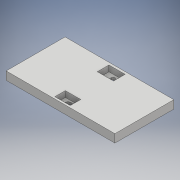
# Autodesk Inventor part: Parte7
Saved by Autodesk Inventor 2017 (Build 210142000, 142)
## iProperties
Part Number: Parte7
Material: Generico
Document SubType Name: Modeling
Designer: Federico
Density: 1 g/cm^3
Appearance: Default
Author: Federico
Autodesk Inventor part; units mm, degrees
ref_plane "YZ Plane" through (0, 0, 0) normal (1, 0, 0) x (0, 1, 0)
ref_plane "XZ Plane" through (0, 0, 0) normal (0, 1, 0) x (-1, 0, 0)
ref_plane "XY Plane" through (0, 0, 0) normal (0, 0, 1) x (1, 0, 0)
sketch "Schizzo1" plane through (0, 0, 0) normal (0, 0, 1) x (1, 0, 0)
  line L0 (-60, 32.5) -> (60, 32.5)
  line L1 (60, 32.5) -> (60, -32.5)
  line L2 (60, -32.5) -> (-60, -32.5)
  line L3 (-60, -32.5) -> (-60, 32.5)
  line L4 (-60, 32.5) -> (60, -32.5) construction
  line L5 (60, 32.5) -> (-60, -32.5) construction
  line L6 (-8.5, -18.7) -> (8.5, -18.7)
  line L7 (8.5, -18.7) -> (8.5, -30.3)
  line L8 (8.5, -30.3) -> (-8.5, -30.3)
  line L9 (-8.5, -30.3) -> (-8.5, -18.7)
  line L10 (-8.5, -18.7) -> (8.5, -30.3) construction
  line L11 (8.5, -18.7) -> (-8.5, -30.3) construction
  line L12 (-12, 12) -> (12, -12) construction
  line L13 (12, 12) -> (-12, -12) construction
  line L14 (-8.95, 29.85) -> (8.95, 29.85)
  line L15 (8.95, 29.85) -> (8.95, 17)
  line L16 (8.95, 17) -> (-8.95, 17)
  line L17 (-8.95, 17) -> (-8.95, 29.85)
  line L18 (-8.95, 29.85) -> (8.95, 17) construction
  line L19 (8.95, 29.85) -> (-8.95, 17) construction
  circle A0 centre (0, -24.5) radius 4.1
  line L20 (0, 25.425) -> (0, 21.425) construction
  line L21 (-2, 25.425) -> (-2, 21.425)
  line L22 (2, 21.425) -> (2, 25.425)
  arc A1 (2, 25.425) -> (-2, 25.425) centre (0, 25.425) ccw
  arc A2 (-2, 21.425) -> (2, 21.425) centre (0, 21.425) ccw
  point P0 (0, 0)
  point P1 (0, 0)
  point P2 (0, 23.425)
  dimension "d0" = 120
  dimension "d1" = 65
  dimension "d2" = 17
  dimension "d3" = 11.6
  dimension "d4" = 24
  dimension "d5" = 24
  dimension "d6" = 17.9
  dimension "d7" = 12.85
  dimension "d8" = 8.2
  dimension "d9" = 2
  dimension "d10" = 4
  constraints: 48 end point, 7 midpoint, 7 parallel, 4 perpendicular, 4 point on circle, 4 tangent, 3 centre point, 3 horizontal
  measures "d0" distance of L1.end L2.end
  measures "d1" distance of L0.end L1.end
  measures "d2" distance of L7.end L8.end
  measures "d3" distance of L6.end L7.end
  measures "d4" distance of L12.end L13.end
  measures "d5" distance of L13.start L12.end
  measures "d6" distance of L16.start L17.start
  measures "d7" distance of L14.end L16.start
  measures "d8" diameter of A0
  measures "d9" distance of point (0, 23.425) L20.end
  measures "d10" diameter of A2
extrude "Estrusione1" add sketch "Schizzo1" along normal blind 9 contours L0 L1 L2 L3
sketch "Schizzo2" plane through (0, 0, 0) normal (0, 0, -1) x (-1, 0, 0)
  line L0 (-60, 32.5) -> (60, 32.5)
  line L1 (60, 32.5) -> (60, -32.5)
  line L2 (60, -32.5) -> (-60, -32.5)
  line L3 (-60, -32.5) -> (-60, 32.5)
  line L4 (-60, 32.5) -> (60, -32.5) construction
  line L5 (60, 32.5) -> (-60, -32.5) construction
  line L6 (-8.95, 17) -> (-8.95, 29.85)
  line L7 (-12, 12) -> (12, -12) construction
  line L8 (12, 12) -> (-12, -12) construction
  line L9 (8.95, 17) -> (-8.95, 17)
  line L10 (-8.95, 29.85) -> (8.95, 29.85)
  line L11 (8.95, 29.85) -> (-8.95, 17) construction
  line L12 (8.95, 29.85) -> (8.95, 17)
  line L13 (-8.95, 29.85) -> (8.95, 17) construction
  line L14 (-8.5, -18.7) -> (8.5, -18.7)
  line L15 (8.5, -18.7) -> (8.5, -30.3)
  line L16 (8.5, -30.3) -> (-8.5, -30.3)
  line L17 (-8.5, -30.3) -> (-8.5, -18.7)
  line L18 (-8.5, -18.7) -> (8.5, -30.3) construction
  line L19 (8.5, -18.7) -> (-8.5, -30.3) construction
  circle A0 centre (0, -24.5) radius 4.1
  line L20 (0, 25.425) -> (0, 21.425) construction
  line L21 (-2, 25.425) -> (-2, 21.425)
  line L22 (2, 21.425) -> (2, 25.425)
  arc A1 (2, 25.425) -> (-2, 25.425) centre (0, 25.425) ccw
  arc A2 (-2, 21.425) -> (2, 21.425) centre (0, 21.425) ccw
  point P0 (0, 0)
  point P1 (0, 0)
  point P2 (0, 0)
  point P3 (0, 23.425)
  dimension "d13" = 120
  dimension "d14" = 65
  dimension "d15" = 17
  dimension "d16" = 11.6
  dimension "d17" = 24
  dimension "d18" = 24
  dimension "d19" = 17.9
  dimension "d20" = 12.85
  dimension "d21" = 8.2
  dimension "d22" = 2
  dimension "d23" = 4
  constraints: 48 end point, 7 midpoint, 7 parallel, 4 perpendicular, 4 point on circle, 4 tangent, 3 centre point, 3 horizontal
  measures "d13" distance of L1.end L2.end
  measures "d14" distance of L0.end L1.end
  measures "d15" distance of L15.end L16.end
  measures "d16" distance of L14.end L15.end
  measures "d17" distance of L7.end L8.end
  measures "d18" distance of L8.start L7.end
  measures "d19" distance of L9.start L6.start
  measures "d20" distance of L10.end L9.start
  measures "d21" diameter of A0
  measures "d22" distance of point (0, 23.425) L20.end
  measures "d23" diameter of A2
extrude "Estrusione2" add sketch "Schizzo2" against normal blind 2.5 contours L6 L10 L12 L9 | L14 L15 L16 L17
